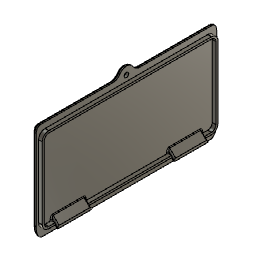
[a]_filter_access_cover (Autodesk Fusion 360 design; units mm, degrees)
Autodesk Fusion 360 part; units mm, degrees
sketch "Sketch1" plane through (0, 0, 0) normal (1, 0, 0) x (0, 1, 0) in component "[a]_filter_access_cover"
  line L0 (-62.4813, -36.2003) -> (62.4813, -36.2003)
  line L1 (67.5678, 36.291) -> (-67.399, -36.2003) construction
  line L2 (-67.5622, 36.2869) -> (67.401, -36.2003) construction
  line L3 (0, 0) -> (0, 50) construction
  arc A0 (4.9336, 39.912) -> (-4.9336, 39.912) centre (0, 36.951) ccw
  line L4 (63.999, 36.9997) -> (10.0782, 36.9997)
  line L5 (-10.0782, 36.9997) -> (-63.999, 36.9997)
  arc A1 (-10.0782, 36.9997) -> (-4.9336, 39.912) centre (-10.0782, 42.9997) ccw
  arc A2 (4.9336, 39.912) -> (10.0782, 36.9997) centre (10.0782, 42.9997) ccw
  line L6 (0, 0) -> (70, 0) construction
  spline S0 degree 3 poles (62.4813, -36.2003) (62.9756, -36.2003) (63.3447, -36.1238) (64.1536, -35.819) (64.589, -35.5423) (65.4299, -34.8113) (65.8191, -34.3263) (66.474, -33.2137) (66.7253, -32.5692) (66.8662, -31.9448) knots 0 0 0 0 0.112438 0.112438 0.263103 0.263103 0.444474 0.444474 0.646408 0.646408 0.646408 0.646408
  line L7 (62.4813, -36.2003) -> (62.9756, -36.2003)
  line L8 (62.9756, -36.2003) -> (63.3447, -36.1238)
  line L9 (63.3447, -36.1238) -> (64.1536, -35.819)
  line L10 (64.1536, -35.819) -> (64.589, -35.5423)
  line L11 (64.589, -35.5423) -> (65.4299, -34.8113)
  line L12 (65.4299, -34.8113) -> (65.8191, -34.3263)
  line L13 (65.8191, -34.3263) -> (66.474, -33.2137)
  line L14 (66.474, -33.2137) -> (66.7253, -32.5692)
  line L15 (66.7253, -32.5692) -> (66.8662, -31.9448)
  arc A3 (66.8662, -31.9448) -> (67.4, -27.1723) centre (45.8, -27.1723) ccw
  arc A4 (-67.4, -27.1723) -> (-66.8662, -31.9448) centre (-45.8, -27.1723) ccw
  spline S1 degree 3 poles (-62.4813, -36.2003) (-62.9756, -36.2003) (-63.3447, -36.1238) (-64.1536, -35.819) (-64.589, -35.5423) (-65.4299, -34.8113) (-65.8191, -34.3263) (-66.474, -33.2137) (-66.7253, -32.5692) (-66.8662, -31.9448) knots 0 0 0 0 0.112438 0.112438 0.263103 0.263103 0.444474 0.444474 0.646408 0.646408 0.646408 0.646408
  line L16 (-62.4813, -36.2003) -> (-62.9756, -36.2003)
  line L17 (-62.9756, -36.2003) -> (-63.3447, -36.1238)
  line L18 (-63.3447, -36.1238) -> (-64.1536, -35.819)
  line L19 (-64.1536, -35.819) -> (-64.589, -35.5423)
  line L20 (-64.589, -35.5423) -> (-65.4299, -34.8113)
  line L21 (-65.4299, -34.8113) -> (-65.8191, -34.3263)
  line L22 (-65.8191, -34.3263) -> (-66.474, -33.2137)
  line L23 (-66.474, -33.2137) -> (-66.7253, -32.5692)
  line L24 (-66.7253, -32.5692) -> (-66.8662, -31.9448)
  ellipse E0 centre (63.9323, 32.5449) end of major axis (64.1013, 36.9977) minor radius 3.4661 (67.4, 32.6306) -> (63.999, 36.9997) ccw
  line L25 (67.4, 32.6306) -> (67.4, -27.1723)
  ellipse E1 centre (-63.9323, 32.5449) end of major axis (-64.1013, 36.9977) minor radius 3.4661 (-63.999, 36.9997) -> (-67.4, 32.6306) ccw
  line L26 (-67.4, 32.6306) -> (-67.4, -27.1723)
  dimension "d3" = 11.508
  dimension "d5" = 6
  dimension "d6" = 6
  dimension "d15" = 21.6
  dimension "d16" = 73.2
  dimension "d18" = 134.8
  constraint horizontal L4
  constraint parallel L0 L4
  constraint coincident L1 L3.start
  constraint coincident L2 L3.start
  constraint coincident L3.start L6.start
  constraint vertical L3
  constraint coincident L3 A0.centre
  constraint collinear L4 L5
  constraint tangent L5 A1
  constraint tangent A0 A1
  constraint tangent A0 A2
  constraint tangent L4 A2
  constraint symmetric L3 L4.start L5.end
  constraint perpendicular L3 L6
  constraint coincident L0.end S0.start
  constraint symmetric L3 L0.end L0.start
  constraint symmetric L3 S0.end A4.end
  constraint symmetric L3 S0 S1
  constraint symmetric L3 A3.end A4.start
  constraint symmetric L3 A3 A4
  constraint coincident S1 L0.start
  constraint symmetric L3 L25.start L26.start
  constraint symmetric L3 E0 E1
  constraint parallel L25 L26
  constraint tangent A3 L25
  constraint tangent E1 L26
  constraint tangent L5 E1
  measures "d3" diameter of A0
  measures "d5" radius of A1
  measures "d6" radius of A2
  measures "d15" radius of A3
  measures "d16" distance of L0 L5
  measures "d18" distance of L25 L26
extrude "Extrude1" add sketch "Sketch1" along normal blind 2.4 contours L0 A0 L4 L5 A1 A2 S0 A3 A4 S1 E0 L25 E1 L26 in component "[a]_filter_access_cover"
sketch "Sketch2" plane through (0, 0, 0) normal (-1, 0, 0) x (0, -1, 0) in component "[a]_filter_access_cover"
  line L0 (63.999, 36.9997) -> (10.0782, 36.9997)
  arc A0 (4.9336, 39.912) -> (10.0782, 36.9997) centre (10.0782, 42.9997) ccw
  arc A1 (4.9336, 39.912) -> (-4.9336, 39.912) centre (0, 36.951) ccw
  arc A2 (-10.0782, 36.9997) -> (-4.9336, 39.912) centre (-10.0782, 42.9997) ccw
  line L1 (-10.0782, 36.9997) -> (-63.999, 36.9997)
  ellipse E0 centre (-63.9323, 32.5449) end of major axis (-64.1013, 36.9977) minor radius 3.4661 (-63.999, 36.9997) -> (-67.4, 32.6306) ccw
  line L2 (-67.4, 32.6306) -> (-67.4, -27.1723)
  arc A3 (-67.4, -27.1723) -> (-66.8662, -31.9448) centre (-45.8, -27.1723) ccw
  spline S0 degree 3 poles (-62.4813, -36.2003) (-62.9756, -36.2003) (-63.3447, -36.1238) (-64.1536, -35.819) (-64.589, -35.5423) (-65.4299, -34.8113) (-65.8191, -34.3263) (-66.474, -33.2137) (-66.7253, -32.5692) (-66.8662, -31.9448) knots 0 0 0 0 0.112438 0.112438 0.263103 0.263103 0.444474 0.444474 0.646408 0.646408 0.646408 0.646408
  line L3 (-62.4813, -36.2003) -> (62.4813, -36.2003)
  spline S1 degree 3 poles (62.4813, -36.2003) (62.9756, -36.2003) (63.3447, -36.1238) (64.1536, -35.819) (64.589, -35.5423) (65.4299, -34.8113) (65.8191, -34.3263) (66.474, -33.2137) (66.7253, -32.5692) (66.8662, -31.9448) knots 0 0 0 0 0.112438 0.112438 0.263103 0.263103 0.444474 0.444474 0.646408 0.646408 0.646408 0.646408
  arc A4 (66.8662, -31.9448) -> (67.4, -27.1723) centre (45.8, -27.1723) ccw
  line L4 (67.4, -27.1723) -> (67.4, 32.6306)
  ellipse E1 centre (63.9323, 32.5449) end of major axis (64.1013, 36.9977) minor radius 3.4661 (67.4, 32.6306) -> (63.999, 36.9997) ccw
  line L5 (56.4, -30.9997) -> (-56.4, -30.9997)
  line L6 (-61.4, -25.9997) -> (-61.4, 25.9997)
  line L7 (-56.4, 30.9997) -> (56.4, 30.9997)
  line L8 (61.4, 25.9997) -> (61.4, -25.9997)
  line L9 (61.4, -30.9997) -> (-61.4, 30.9997) construction
  line L10 (-61.4, -30.9997) -> (61.4, 30.9997) construction
  arc A5 (-56.4, 30.9997) -> (-61.4, 25.9997) centre (-56.4, 25.9997) ccw
  arc A6 (56.4, -30.9997) -> (61.4, -25.9997) centre (56.4, -25.9997) ccw
  arc A7 (-61.4, -25.9997) -> (-56.4, -30.9997) centre (-56.4, -25.9997) ccw
  arc A8 (61.4, 25.9997) -> (56.4, 30.9997) centre (56.4, 25.9997) ccw
  arc A9 (59.4, 25.9997) -> (56.4, 28.9997) centre (56.4, 25.9997) ccw
  line L11 (-56.4, 28.9997) -> (56.4, 28.9997)
  arc A10 (-56.4, 28.9997) -> (-59.4, 25.9997) centre (-56.4, 25.9997) ccw
  line L12 (-59.4, -25.9997) -> (-59.4, 25.9997)
  arc A11 (-59.4, -25.9997) -> (-56.4, -28.9997) centre (-56.4, -25.9997) ccw
  line L13 (56.4, -28.9997) -> (-56.4, -28.9997)
  arc A12 (56.4, -28.9997) -> (59.4, -25.9997) centre (56.4, -25.9997) ccw
  line L14 (59.4, 25.9997) -> (59.4, -25.9997)
  line L15 (-12.6908, 0.3342) -> (-7.2507, 0.3342)
  line L16 (-7.2507, 0.3342) -> (0.1907, 11.6542)
  line L17 (0.1907, 11.6542) -> (-5.2499, 11.6542)
  line L18 (-5.2499, 11.6542) -> (-12.6908, 0.3342)
  line L19 (-4.6684, -10.9853) -> (10.2144, 11.6542)
  line L20 (10.2144, 11.6542) -> (4.7747, 11.6542)
  line L21 (4.7747, 11.6542) -> (-10.1076, -10.9853)
  line L22 (-10.1076, -10.9853) -> (-4.6684, -10.9853)
  line L23 (12.7966, 0.3342) -> (7.356, 0.3342)
  line L24 (7.356, 0.3342) -> (-0.0839, -10.9853)
  line L25 (-0.0839, -10.9853) -> (5.3557, -10.9853)
  line L26 (5.3557, -10.9853) -> (12.7966, 0.3342)
  dimension "d21" = 6
  dimension "d22" = 6
  dimension "d23" = 5
  dimension "d24" = 5
  dimension "d25" = 2
  constraint horizontal L5
  constraint perpendicular L5 L6
  constraint parallel L5 L7
  constraint parallel L6 L8
  constraint coincident L9 origin
  constraint coincident L10 origin
  constraint coincident L9.end L6
  constraint coincident L9.end L7
  constraint tangent L6 A5
  constraint tangent L7 A5
  constraint coincident L9.start L5
  constraint coincident L9.start L8
  constraint tangent L5 A6
  constraint tangent L8 A6
  constraint equal A5 A6
  constraint coincident L10.start L5
  constraint coincident L10.start L6
  constraint tangent L5 A7
  constraint tangent L6 A7
  constraint equal A5 A7
  constraint coincident L10.end L7
  constraint coincident L10.end L8
  constraint tangent L7 A8
  constraint tangent L8 A8
  measures "d21" distance of L1 L7
  measures "d22" distance of L2 L6
  measures "d23" radius of A5
  measures "d24" radius of A8
extrude "Extrude2" cut sketch "Sketch2" against normal blind 1 contours L5 L6 L7 L8 A5 A6 A7 A8 | L15 L16 L17 L18 | L19 L20 L21 L22 | L23 L24 L25 L26 in component "[a]_filter_access_cover"
sketch "Sketch3" plane through (0, 0, 0) normal (-1, 0, 0) x (0, -1, 0) in component "[a]_filter_access_cover"
  line L0 (63.999, 36.9997) -> (10.0782, 36.9997)
  arc A0 (4.9336, 39.912) -> (10.0782, 36.9997) centre (10.0782, 42.9997) ccw
  arc A1 (4.9336, 39.912) -> (-4.9336, 39.912) centre (0, 36.951) ccw
  arc A2 (-10.0782, 36.9997) -> (-4.9336, 39.912) centre (-10.0782, 42.9997) ccw
  line L1 (-10.0782, 36.9997) -> (-63.999, 36.9997)
  ellipse E0 centre (-63.9323, 32.5449) end of major axis (-64.1013, 36.9977) minor radius 3.4661 (-63.999, 36.9997) -> (-67.4, 32.6306) ccw
  line L2 (-67.4, 32.6306) -> (-67.4, -27.1723)
  arc A3 (-67.4, -27.1723) -> (-66.8662, -31.9448) centre (-45.8, -27.1723) ccw
  spline S0 degree 3 poles (-62.4813, -36.2003) (-62.9756, -36.2003) (-63.3447, -36.1238) (-64.1536, -35.819) (-64.589, -35.5423) (-65.4299, -34.8113) (-65.8191, -34.3263) (-66.474, -33.2137) (-66.7253, -32.5692) (-66.8662, -31.9448) knots 0 0 0 0 0.112438 0.112438 0.263103 0.263103 0.444474 0.444474 0.646408 0.646408 0.646408 0.646408
  line L3 (-62.4813, -36.2003) -> (62.4813, -36.2003)
  spline S1 degree 3 poles (62.4813, -36.2003) (62.9756, -36.2003) (63.3447, -36.1238) (64.1536, -35.819) (64.589, -35.5423) (65.4299, -34.8113) (65.8191, -34.3263) (66.474, -33.2137) (66.7253, -32.5692) (66.8662, -31.9448) knots 0 0 0 0 0.112438 0.112438 0.263103 0.263103 0.444474 0.444474 0.646408 0.646408 0.646408 0.646408
  arc A4 (66.8662, -31.9448) -> (67.4, -27.1723) centre (45.8, -27.1723) ccw
  line L4 (67.4, -27.1723) -> (67.4, 32.6306)
  ellipse E1 centre (63.9323, 32.5449) end of major axis (64.1013, 36.9977) minor radius 3.4661 (67.4, 32.6306) -> (63.999, 36.9997) ccw
  line L5 (61.4, 25.9997) -> (61.4, -25.9997)
  arc A5 (56.4, -30.9997) -> (61.4, -25.9997) centre (56.4, -25.9997) ccw
  line L6 (56.4, -30.9997) -> (-56.4, -30.9997)
  arc A6 (-61.4, -25.9997) -> (-56.4, -30.9997) centre (-56.4, -25.9997) ccw
  line L7 (-61.4, -25.9997) -> (-61.4, 25.9997)
  arc A7 (-56.4, 30.9997) -> (-61.4, 25.9997) centre (-56.4, 25.9997) ccw
  line L8 (-56.4, 30.9997) -> (56.4, 30.9997)
  arc A8 (61.4, 25.9997) -> (56.4, 30.9997) centre (56.4, 25.9997) ccw
hole "Hole1" at (0, 0, 36.951) direction (1, 0, 0) diameter 3.4 end through all in component "[a]_filter_access_cover"
sketch "Sketch1 (2)" plane through (2.4, 0, 0) normal (1, 0, 0) x (0, 1, 0) in component "[a]_filter_access_cover"
  circle A0 centre (0, 36.951) radius 1.7
  line L0 (-10.0782, 36.9997) -> (-63.999, 36.9997)
  ellipse E0 centre (-63.9323, 32.5449) end of major axis (-64.1013, 36.9977) minor radius 3.4661 (-63.999, 36.9997) -> (-67.4, 32.6306) ccw
  line L1 (-67.4, 32.6306) -> (-67.4, -27.1723)
  arc A1 (-67.4, -27.1723) -> (-66.8662, -31.9448) centre (-45.8, -27.1723) ccw
  spline S0 degree 3 poles (-66.8662, -31.9448) (-66.7253, -32.5692) (-66.474, -33.2137) (-65.8191, -34.3263) (-65.4299, -34.8113) (-64.589, -35.5423) (-64.1536, -35.819) (-63.3447, -36.1238) (-62.9756, -36.2003) (-62.4813, -36.2003) knots -0.646408 -0.646408 -0.646408 -0.646408 -0.444474 -0.444474 -0.263103 -0.263103 -0.112438 -0.112438 0 0 0 0
  line L2 (-62.4813, -36.2003) -> (62.4813, -36.2003)
  spline S1 degree 3 poles (62.4813, -36.2003) (62.9756, -36.2003) (63.3447, -36.1238) (64.1536, -35.819) (64.589, -35.5423) (65.4299, -34.8113) (65.8191, -34.3263) (66.474, -33.2137) (66.7253, -32.5692) (66.8662, -31.9448) knots 0 0 0 0 0.112438 0.112438 0.263103 0.263103 0.444474 0.444474 0.646408 0.646408 0.646408 0.646408
  arc A2 (66.8662, -31.9448) -> (67.4, -27.1723) centre (45.8, -27.1723) ccw
  line L3 (67.4, -27.1723) -> (67.4, 32.6306)
  ellipse E1 centre (63.9323, 32.5449) end of major axis (64.1013, 36.9977) minor radius 3.4661 (67.4, 32.6306) -> (63.999, 36.9997) ccw
  line L4 (63.999, 36.9997) -> (10.0782, 36.9997)
  arc A3 (4.9336, 39.912) -> (10.0782, 36.9997) centre (10.0782, 42.9997) ccw
  arc A4 (4.9336, 39.912) -> (-4.9336, 39.912) centre (0, 36.951) ccw
  arc A5 (-10.0782, 36.9997) -> (-4.9336, 39.912) centre (-10.0782, 42.9997) ccw
  line L5 (60.8, -30.7003) -> (-60.8, -30.7003)
  line L6 (-65.6, -25.9003) -> (-65.6, 27.8997)
  line L7 (-60.8, 32.6997) -> (60.8, 32.6997)
  line L8 (65.6, 27.8997) -> (65.6, -25.9003)
  line L9 (65.6, -30.7003) -> (-65.6, 32.6997) construction
  line L10 (-65.6, -30.7003) -> (65.6, 32.6997) construction
  arc A6 (-60.8, 32.6997) -> (-65.6, 27.8997) centre (-60.8, 27.8997) ccw
  arc A7 (65.6, 27.8997) -> (60.8, 32.6997) centre (60.8, 27.8997) ccw
  arc A8 (60.8, -30.7003) -> (65.6, -25.9003) centre (60.8, -25.9003) ccw
  arc A9 (-65.6, -25.9003) -> (-60.8, -30.7003) centre (-60.8, -25.9003) ccw
  arc A10 (64.1, 27.8997) -> (60.8, 31.1997) centre (60.8, 27.8997) ccw
  line L11 (-60.8, 31.1997) -> (60.8, 31.1997)
  arc A11 (-60.8, 31.1997) -> (-64.1, 27.8997) centre (-60.8, 27.8997) ccw
  line L12 (-64.1, -25.9003) -> (-64.1, 27.8997)
  arc A12 (-64.1, -25.9003) -> (-60.8, -29.2003) centre (-60.8, -25.9003) ccw
  line L13 (60.8, -29.2003) -> (-60.8, -29.2003)
  arc A13 (60.8, -29.2003) -> (64.1, -25.9003) centre (60.8, -25.9003) ccw
  line L14 (64.1, 27.8997) -> (64.1, -25.9003)
  line L15 (0, 0) -> (0, 50) construction
  line L16 (-56.3, -29.2003) -> (-31.3, -29.2003)
  line L17 (-31.3, -29.2003) -> (-31.3, -27.2003)
  line L18 (-31.3, -27.2003) -> (-56.3, -27.2003)
  line L19 (-56.3, -27.2003) -> (-56.3, -29.2003)
  line L20 (31.3, -27.2003) -> (56.3, -27.2003)
  line L21 (56.3, -27.2003) -> (56.3, -29.2003)
  line L22 (31.3, -29.2003) -> (31.3, -27.2003)
  dimension "d32" = 4.3
  dimension "d33" = 1.8
  dimension "d35" = 1.8
  dimension "d36" = 4.8
  dimension "d37" = 4.8
  dimension "d38" = 4.8
  dimension "d39" = 4.8
  dimension "d40" = 1.5
  dimension "d43" = 25
  dimension "d44" = 2
  dimension "d45" = 31.3
  constraint horizontal L5
  constraint perpendicular L5 L6
  constraint parallel L5 L7
  constraint parallel L6 L8
  constraint coincident L9.end L6
  constraint coincident L9.end L7
  constraint tangent L6 A6
  constraint tangent L7 A6
  constraint coincident L10.end L7
  constraint coincident L10.end L8
  constraint tangent L7 A7
  constraint tangent L8 A7
  constraint coincident L9.start L5
  constraint coincident L9.start L8
  constraint tangent L5 A8
  constraint tangent L8 A8
  constraint coincident L10.start L6
  constraint coincident L10.start L5
  constraint tangent L6 A9
  constraint tangent L5 A9
  constraint coincident L15.start origin
  constraint vertical L15
  constraint horizontal L16
  constraint vertical L17
  constraint horizontal L18
  constraint vertical L19
  constraint coincident L13 L16.start
  constraint symmetric L15 L16.start L21.end
  constraint symmetric L15 L16.end L22.start
  constraint symmetric L15 L17.end L20.start
  constraint symmetric L15 L18.end L20.end
  measures "d32" distance of L0 L7
  measures "d33" distance of L1 L6
  measures "d35" distance of L3 L8
  measures "d36" radius of A6
  measures "d37" radius of A7
  measures "d38" radius of A8
  measures "d39" radius of A9
  measures "d43" distance of L16.start L16.end
  measures "d44" distance of L16.start L18.end
  measures "d45" distance of L15 L16.end
extrude "Extrude3" add sketch "Sketch1 (2)" along normal blind 2.8 contours L5 L6 L7 L8 A6 A7 A8 A9 in component "[a]_filter_access_cover"
sketch "Sketch5" plane through (0, 0, 0) normal (0, 1, 0) x (1, 0, 0) in component "[a]_filter_access_cover"
  line L0 (2.4, 30.7003) -> (5.2, 30.7003)
  line L1 (5.2, 25.9003) -> (5.2, 30.7003)
  line L2 (2.4, 25.9003) -> (2.4, 29.2003)
  line L3 (2.4, 25.9003) -> (2.4, -27.8997)
  line L4 (2.4, -31.1997) -> (2.4, -27.8997)
  line L5 (2.4, -31.1997) -> (2.4, -27.8997)
  line L6 (2.4, -27.8997) -> (2.4, 25.9003)
  line L7 (2.4, 25.9003) -> (2.4, 29.2003)
  line L8 (5.2, 30.7003) -> (2.4, 27.9003)
  line L9 (5.2, 30.7003) -> (9.1598, 30.7003) construction
  line L10 (5.2, 30.7003) -> (7.2, 32.7003)
  line L11 (7.2, 32.7003) -> (7.2, 30.4003)
  line L12 (7.2, 30.4003) -> (2.4, 25.9003)
  line L13 (2.4, 25.9003) -> (2.4, 27.9003)
  line L14 (6.75, 32.2503) -> (7.2, 32.2503)
  line L15 (5.2, 30.7003) -> (2.4, 30.7003)
  line L16 (2.4, 27.9003) -> (2.4, 30.7003)
  dimension "d59" = 135
  dimension "d60" = 2
  dimension "d61" = 2.3
  dimension "d62" = 1.85
  constraint horizontal L9
  constraint coincident L0.end L1.end
  constraint parallel L8 L10
  constraint perpendicular L9 L11
  constraint coincident L2.start L3.start
  constraint coincident L10 L14.start
  constraint coincident L11 L14.end
  constraint perpendicular L11 L14
  constraint coincident L0.start L15.end
  constraint perpendicular L15 L16
  measures "d59" angle of L8 L9
  measures "d60" horizontal distance of L0.end L10.end
  measures "d61" distance of L10.end L11.end
  measures "d62" distance of L11.end L14.end
extrude "Extrude5" add sketch "Sketch5" along normal blind 25 from surface at 31 contours L0 L2 L7 L8 L15 L16 | L1 L10 L11 L12 L14 | L1 L2 L7 L8 L12 L13 in component "[a]_filter_access_cover"
extrude "Extrude6" add sketch "Sketch5" against normal blind 25 from surface at -31 contours L0 L2 L7 L8 L15 L16 | L1 L10 L11 L12 L14 | L1 L2 L7 L8 L12 L13 in component "[a]_filter_access_cover"
fillet "Fillet2" radius 1 10 edges at (4.8, -56, -28.1503) (4.8, -31, -28.1503) (4.8, 31, -28.1503) (4.8, 56, -28.1503) (2.4, -56, -27.5503) (2.4, -43.5, -25.9003) (2.4, -31, -27.5503) (2.4, 56, -27.5503) (2.4, 43.5, -25.9003) (2.4, 31, -27.5503) in component "[a]_filter_access_cover"
chamfer "Chamfer2" distance 1 angle 45 14 edges at (0, 37.0386, 36.9997) (0, 7.1223, 37.7783) (0, 0, 42.705) (0, -7.1223, 37.7783) (0, -37.0386, 36.9997) (0, -66.4078, 35.7251) (0, -67.4, 2.7292) (0, -67.2661, -29.5734) (0, -65.4037, -34.7871) (0, 0, -36.2003) (0, 65.4037, -34.7871) (0, 67.2661, -29.5734) (0, 67.4, 2.7292) (0, 66.4078, 35.7251) in component "[a]_filter_access_cover"
fillet "Fillet3" radius 1 14 edges at (1, 67.4, 2.7292) (1, 67.2661, -29.5734) (1, 65.4037, -34.7871) (1, 0, -36.2003) (1, -65.4037, -34.7871) (1, -67.2661, -29.5734) (1, -67.4, 2.7292) (1, -66.4078, 35.7251) (1, -37.0386, 36.9997) (1, -7.1223, 37.7783) (1, 0, 42.705) (1, 7.1223, 37.7783) (1, 37.0386, 36.9997) (1, 66.4078, 35.7251) in component "[a]_filter_access_cover"
chamfer "Chamfer3" distance 0.4 angle 45 1 edges at (0, 1.585, 37.5657) in component "[a]_filter_access_cover"
component "[a]_filter_access_cover" placed x (1, 0, 0) y (0, 1, 0) z (0, 0, 1) at (0, 0, 0)
equation "d3 = 5.754 mm * 2"
